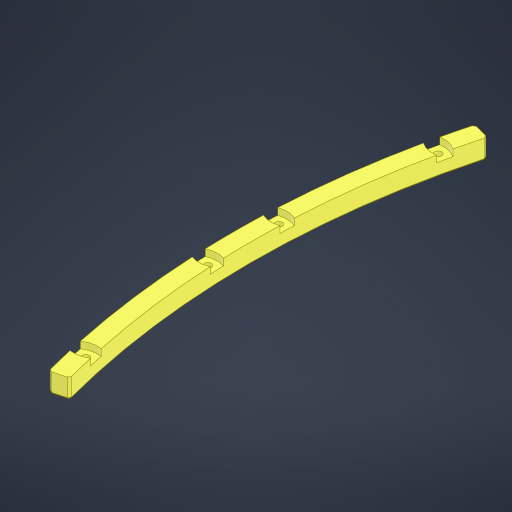
# Autodesk Inventor part: LED-Ring_Connector_v2
Saved by Autodesk Inventor 2023.2 (Build 272271030, 271C)
## iProperties
Created: 2023-02-19
Part Number: LED-Ring_Connector_v2
Material: Generisch
Document SubType Name: Modeling
Designer: Stefan
Mass: 12.3659 g
Surface Area: 65.418 cm^2
Volume: 12.3659 cm^3
Density: 1 g/cm^3
Appearance: Glatt - Gelb
Author: Stefan
Autodesk Inventor part; units mm, degrees
ref_plane "YZ Plane" through (0, 0, 0) normal (1, 0, 0) x (0, 1, 0)
ref_plane "XZ Plane" through (0, 0, 0) normal (0, 1, 0) x (-1, 0, 0)
ref_plane "XY Plane" through (0, 0, 0) normal (0, 0, 1) x (1, 0, 0)
sketch "Skizze1" plane through (0, 0, 0) normal (0, 1, 0) x (-1, 0, 0)
  arc A0 (349.7617, -93.7184) -> (349.7617, 93.7184) centre (0, 0) ccw
  arc A1 (357.296, -95.7372) -> (357.296, 95.7372) centre (0, 0) ccw
  line L0 (357.296, 95.7372) -> (0, 0) construction
  line L1 (0, 0) -> (357.296, -95.7372) construction
  line L2 (444.782, 0) -> (-74.1303, 0) construction
  line L3 (357.296, 95.7372) -> (349.7617, 93.7184)
  line L4 (357.296, -95.7372) -> (349.7617, -93.7184)
  line L5 (361.1319, 80.061) -> (0, 0) construction
  line L6 (369.5479, 16.1348) -> (0, 0) construction
  line L7 (369.5479, -16.1348) -> (0, 0) construction
  line L8 (361.1319, -80.061) -> (0, 0) construction
  arc A2 (353.5289, -94.7278) -> (353.5289, 94.7278) centre (0, 0) ccw construction
  circle A3 centre (357.3243, 79.2169) radius 1.6
  circle A4 centre (365.6516, 15.9647) radius 1.6
  circle A5 centre (365.6516, -15.9647) radius 1.6
  circle A6 centre (357.3243, -79.2169) radius 1.6
  circle A7 centre (357.3243, 79.2169) radius 3
  circle A8 centre (365.6516, 15.9647) radius 3
  circle A9 centre (365.6516, -15.9647) radius 3
  circle A10 centre (357.3243, -79.2169) radius 3
  arc A11 (360.4527, 83.0652) -> (352.8301, 81.4083) centre (358.5974, 73.2389) ccw
  arc A12 (354.1773, 75.3315) -> (361.786, 77.0512) centre (355.9517, 85.1728) ccw
  arc A13 (369.4008, 19.2113) -> (361.6062, 18.9032) centre (365.8673, 9.8564) ccw
  arc A14 (361.8777, 12.6848) -> (369.6695, 13.0572) centre (365.3341, 22.0685) ccw
  arc A15 (369.6695, -13.0572) -> (361.8777, -12.6848) centre (365.3341, -22.0685) ccw
  arc A16 (361.786, -77.0512) -> (354.1773, -75.3315) centre (355.9517, -85.1728) ccw
  arc A17 (352.8301, -81.4083) -> (360.4527, -83.0652) centre (358.5974, -73.2389) ccw
  arc A18 (361.6062, -18.9032) -> (369.4008, -19.2113) centre (365.8673, -9.8564) ccw
  circle A19 centre (357.3243, -79.2169) radius 5 construction
  circle A20 centre (365.6516, -15.9647) radius 5 construction
  circle A21 centre (365.6516, 15.9647) radius 5 construction
  circle A22 centre (357.3243, 79.2169) radius 5 construction
  dimension "d1" = 7.8
  dimension "d18" = 366
  dimension "d19" = 10
  dimension "d2" = 30
  dimension "d4" = 10
  dimension "d5" = 5
  dimension "d6" = 10
  dimension "d7" = 3.2
  dimension "d8" = 6
  dimension "d17" = 10
  constraints: 16 centre point, 16 end point, 16 point on circle, 9 coincident, 9 equal radius, 6 point on line, 2 collinear, 2 midpoint, 62 other
  measures "d2" angle of L1 L0
  measures "d4" angle of L6 L5
  measures "d5" angle of L7 L6
  measures "d6" angle of L8 L7
  measures "d7" diameter of A3
  measures "d8" diameter of A7
  measures "d17" radius of A11
extrude "Extrusion1" add sketch "Skizze1" against normal blind 6 contours A0 A17 A1 L4 | A0 A16 A1 A17 | A0 A18 A1 A16 | A0 A15 A1 A18 | A0 A14 A1 A15 | A0 A13 A1 A14 | A0 A12 A1 A13 | A0 A11 A1 A12 | A0 L3 A1 A11 | A7 | A8 | A9 | A10
extrude "Extrusion2" add sketch "Skizze1" along normal blind 3 contours A0 A17 A1 L4 | A0 A18 A1 A16 | A0 A14 A1 A15 | A0 A12 A1 A13 | A0 L3 A1 A11
chamfer "Fase1" distance 1 angle 45 8 edges at (-362.1, -6, 0) (-349.7617, -1.5, 93.7184) (-357.296, -1.5, 95.7372) (-349.7617, -1.5, -93.7184) (-357.296, -1.5, -95.7372) (-369.9, -6, 0) (-353.5289, -6, -94.7278) (-353.5289, -6, 94.7278)
